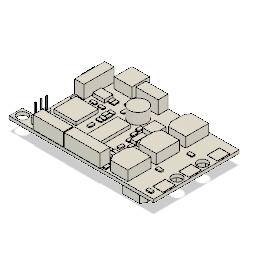
DIY_OneWheel_Frame (Autodesk Fusion 360 archive; units mm, degrees)
design "VESC-Fusion360"
Autodesk Fusion 360 part; units mm, degrees
sketch "Skizze1" plane through (0, 0, 0) normal (0, 1, 0) x (1, 0, 0)
  line L0 (65, 0) -> (65, -38.5) construction
  line L1 (65, -38.5) -> (0, -38.5) construction
  line L2 (6.3179, -1.8001) -> (10.6239, -1.8001)
  line L3 (10.6239, -1.8001) -> (10.6239, -15.3888)
  line L4 (10.6239, -15.3888) -> (6.3179, -15.3888)
  line L5 (6.3179, -15.3888) -> (6.3179, -1.8001)
  line L6 (16.7653, -8.6827) -> (18.1771, -8.6827)
  line L7 (18.1771, -8.6827) -> (18.1771, -11.0828)
  line L8 (18.1771, -11.0828) -> (16.7653, -11.0828)
  line L9 (16.7653, -11.0828) -> (16.7653, -8.6827)
  line L10 (18.3183, -8.6827) -> (19.7301, -8.6827)
  line L11 (19.7301, -8.6827) -> (19.7301, -11.0828)
  line L12 (19.7301, -11.0828) -> (18.3183, -11.0828)
  line L13 (18.3183, -11.0828) -> (18.3183, -8.6827)
  line L14 (21.8126, -6.2826) -> (23.2244, -6.2826)
  line L15 (23.2244, -6.2826) -> (23.2244, -8.6827)
  line L16 (23.2244, -8.6827) -> (21.8126, -8.6827)
  line L17 (21.8126, -8.6827) -> (21.8126, -6.2826)
  line L18 (23.9303, -7.412) -> (25.3421, -7.412)
  line L19 (25.3421, -7.412) -> (25.3421, -9.8121)
  line L20 (25.3421, -9.8121) -> (23.9303, -9.8121)
  line L21 (23.9303, -9.8121) -> (23.9303, -7.412)
  line L22 (23.9303, -9.9533) -> (25.3421, -9.9533)
  line L23 (25.3421, -9.9533) -> (25.3421, -12.3534)
  line L24 (25.3421, -12.3534) -> (23.9303, -12.3534)
  line L25 (23.9303, -12.3534) -> (23.9303, -9.9533)
  line L26 (12.8475, -13.8711) -> (15.2476, -13.8711)
  line L27 (15.2476, -13.8711) -> (15.2476, -15.177)
  line L28 (15.2476, -15.177) -> (12.8475, -15.177)
  line L29 (12.8475, -15.177) -> (12.8475, -13.8711)
  line L30 (16.5536, -13.9417) -> (18.9536, -13.9417)
  line L31 (18.9536, -13.9417) -> (18.9536, -15.2476)
  line L32 (18.9536, -15.2476) -> (16.5536, -15.2476)
  line L33 (16.5536, -15.2476) -> (16.5536, -13.9417)
  line L34 (20.8596, -13.8358) -> (23.2597, -13.8358)
  line L35 (23.2597, -13.8358) -> (23.2597, -15.1417)
  line L36 (23.2597, -15.1417) -> (20.8596, -15.1417)
  line L37 (20.8596, -15.1417) -> (20.8596, -13.8358)
  line L38 (20.6125, -15.2829) -> (22.0243, -15.2829)
  line L39 (22.0243, -15.2829) -> (22.0243, -17.683)
  line L40 (22.0243, -17.683) -> (20.6125, -17.683)
  line L41 (20.6125, -17.683) -> (20.6125, -15.2829)
  line L42 (22.2008, -15.2829) -> (23.5067, -15.2829)
  line L43 (23.5067, -15.2829) -> (23.5067, -17.683)
  line L44 (23.5067, -17.683) -> (22.2008, -17.683)
  line L45 (22.2008, -17.683) -> (22.2008, -15.2829)
  line L46 (21.1067, -17.8242) -> (23.5067, -17.8242)
  line L47 (23.5067, -17.8242) -> (23.5067, -19.236)
  line L48 (23.5067, -19.236) -> (21.1067, -19.236)
  line L49 (21.1067, -19.236) -> (21.1067, -17.8242)
  line L50 (21.142, -19.4125) -> (23.542, -19.4125)
  line L51 (23.542, -19.4125) -> (23.542, -20.7184)
  line L52 (23.542, -20.7184) -> (21.142, -20.7184)
  line L53 (21.142, -20.7184) -> (21.142, -19.4125)
  line L54 (21.6714, -22.8008) -> (22.9773, -22.8008)
  line L55 (22.9773, -22.8008) -> (22.9773, -25.2009)
  line L56 (22.9773, -25.2009) -> (21.6714, -25.2009)
  line L57 (21.6714, -25.2009) -> (21.6714, -22.8008)
  line L58 (7.2003, -15.6712) -> (8.5062, -15.6712)
  line L59 (8.5062, -15.6712) -> (8.5062, -18.0713)
  line L60 (8.5062, -18.0713) -> (7.2003, -18.0713)
  line L61 (7.2003, -18.0713) -> (7.2003, -15.6712)
  line L62 (17.683, -29.1893) -> (20.0831, -29.1893)
  line L63 (20.0831, -29.1893) -> (20.0831, -30.4952)
  line L64 (20.0831, -30.4952) -> (17.683, -30.4952)
  line L65 (17.683, -30.4952) -> (17.683, -29.1893)
  line L66 (22.4479, -29.9305) -> (23.7538, -29.9305)
  line L67 (23.7538, -29.9305) -> (23.7538, -32.3306)
  line L68 (23.7538, -32.3306) -> (22.4479, -32.3306)
  line L69 (22.4479, -32.3306) -> (22.4479, -29.9305)
  line L70 (14.7535, -32.5777) -> (17.1536, -32.5777)
  line L71 (17.1536, -32.5777) -> (17.1536, -33.9895)
  line L72 (17.1536, -33.9895) -> (14.7535, -33.9895)
  line L73 (14.7535, -33.9895) -> (14.7535, -32.5777)
  line L74 (17.33, -32.613) -> (19.7301, -32.613)
  line L75 (19.7301, -32.613) -> (19.7301, -33.9189)
  line L76 (19.7301, -33.9189) -> (17.33, -33.9189)
  line L77 (17.33, -33.9189) -> (17.33, -32.613)
  line L78 (26.7892, -31.3776) -> (31.8718, -31.3776)
  line L79 (31.8718, -31.3776) -> (31.8718, -33.6718)
  line L80 (31.8718, -33.6718) -> (26.7892, -33.6718)
  line L81 (26.7892, -33.6718) -> (26.7892, -31.3776)
  line L82 (35.6484, -28.5187) -> (36.9543, -28.5187)
  line L83 (36.9543, -28.5187) -> (36.9543, -30.9188)
  line L84 (36.9543, -30.9188) -> (35.6484, -30.9188)
  line L85 (35.6484, -30.9188) -> (35.6484, -28.5187)
  line L86 (35.6484, -31.307) -> (36.9543, -31.307)
  line L87 (36.9543, -31.307) -> (36.9543, -33.7071)
  line L88 (36.9543, -33.7071) -> (35.6484, -33.7071)
  line L89 (35.6484, -33.7071) -> (35.6484, -31.307)
  line L90 (37.1308, -28.1304) -> (39.5309, -28.1304)
  line L91 (39.5309, -28.1304) -> (39.5309, -29.5423)
  line L92 (39.5309, -29.5423) -> (37.1308, -29.5423)
  line L93 (37.1308, -29.5423) -> (37.1308, -28.1304)
  line L94 (37.1308, -29.6482) -> (39.5309, -29.6482)
  line L95 (39.5309, -29.6482) -> (39.5309, -31.06)
  line L96 (39.5309, -31.06) -> (37.1308, -31.06)
  line L97 (37.1308, -31.06) -> (37.1308, -29.6482)
  line L98 (37.1308, -31.1659) -> (39.5309, -31.1659)
  line L99 (39.5309, -31.1659) -> (39.5309, -32.5777)
  line L100 (39.5309, -32.5777) -> (37.1308, -32.5777)
  line L101 (37.1308, -32.5777) -> (37.1308, -31.1659)
  line L102 (37.1308, -32.7189) -> (39.5662, -32.7189)
  line L103 (39.5662, -32.7189) -> (39.5662, -34.1307)
  line L104 (39.5662, -34.1307) -> (37.1308, -34.1307)
  line L105 (37.1308, -34.1307) -> (37.1308, -32.7189)
  line L106 (41.4368, -35.366) -> (42.8486, -35.366)
  line L107 (42.8486, -35.366) -> (42.8486, -37.7661)
  line L108 (42.8486, -37.7661) -> (41.4368, -37.7661)
  line L109 (41.4368, -37.7661) -> (41.4368, -35.366)
  line L110 (36.8131, -24.4244) -> (38.1191, -24.4244)
  line L111 (38.1191, -24.4244) -> (38.1191, -26.8245)
  line L112 (38.1191, -26.8245) -> (36.8131, -26.8245)
  line L113 (36.8131, -26.8245) -> (36.8131, -24.4244)
  line L114 (38.9661, -22.0243) -> (40.2721, -22.0243)
  line L115 (40.2721, -22.0243) -> (40.2721, -24.4244)
  line L116 (40.2721, -24.4244) -> (38.9661, -24.4244)
  line L117 (38.9661, -24.4244) -> (38.9661, -22.0243)
  line L118 (36.1778, -19.7654) -> (37.4837, -19.7654)
  line L119 (37.4837, -19.7654) -> (37.4837, -22.1655)
  line L120 (37.4837, -22.1655) -> (36.1778, -22.1655)
  line L121 (36.1778, -22.1655) -> (36.1778, -19.7654)
  line L122 (34.9072, -16.6947) -> (36.2131, -16.6947)
  line L123 (36.2131, -16.6947) -> (36.2131, -19.0948)
  line L124 (36.2131, -19.0948) -> (34.9072, -19.0948)
  line L125 (34.9072, -19.0948) -> (34.9072, -16.6947)
  line L126 (34.0954, -13.377) -> (35.5072, -13.377)
  line L127 (35.5072, -13.377) -> (35.5072, -15.7771)
  line L128 (35.5072, -15.7771) -> (34.0954, -15.7771)
  line L129 (34.0954, -15.7771) -> (34.0954, -13.377)
  line L130 (37.8367, -16.5183) -> (40.1309, -16.5183)
  line L131 (40.1309, -16.5183) -> (40.1309, -21.6008)
  line L132 (40.1309, -21.6008) -> (37.8367, -21.6008)
  line L133 (37.8367, -21.6008) -> (37.8367, -16.5183)
  line L134 (40.378, -16.5183) -> (42.6722, -16.5183)
  line L135 (42.6722, -16.5183) -> (42.6722, -21.6008)
  line L136 (42.6722, -21.6008) -> (40.378, -21.6008)
  line L137 (40.378, -21.6008) -> (40.378, -16.5183)
  line L138 (55.0609, -12.2475) -> (57.4609, -12.2475)
  line L139 (57.4609, -12.2475) -> (57.4609, -13.6593)
  line L140 (57.4609, -13.6593) -> (55.0609, -13.6593)
  line L141 (55.0609, -13.6593) -> (55.0609, -12.2475)
  line L142 (53.8961, -25.2009) -> (56.2962, -25.2009)
  line L143 (56.2962, -25.2009) -> (56.2962, -26.6127)
  line L144 (56.2962, -26.6127) -> (53.8961, -26.6127)
  line L145 (53.8961, -26.6127) -> (53.8961, -25.2009)
  line L146 (60.0022, -35.6131) -> (62.4023, -35.6131)
  line L147 (62.4023, -35.6131) -> (62.4023, -37.0249)
  line L148 (62.4023, -37.0249) -> (60.0022, -37.0249)
  line L149 (60.0022, -37.0249) -> (60.0022, -35.6131)
  line L150 (11.3987, -31.323) -> (13.0958, -33.0201)
  line L151 (13.0958, -33.0201) -> (12.1724, -33.9435)
  line L152 (12.1724, -33.9435) -> (10.4753, -32.2464)
  line L153 (10.4753, -32.2464) -> (11.3987, -31.323)
  circle A0 centre (3.0001, -3.0001) radius 2.2942
  circle A1 centre (3.0001, -35.5072) radius 2.2942
  circle A2 centre (62.0493, -25.0245) radius 2.2942
  circle A3 centre (62.0493, -13.5181) radius 2.2942
  line L154 (59.9316, -16.483) -> (64.52, -16.483)
  line L155 (64.52, -16.483) -> (64.52, -22.0949)
  line L156 (64.52, -22.0949) -> (59.9316, -22.0949)
  line L157 (59.9316, -22.0949) -> (59.9316, -16.483)
  line L158 (59.9316, -3.7766) -> (64.52, -3.7766)
  line L159 (64.52, -3.7766) -> (64.52, -9.3886)
  line L160 (64.52, -9.3886) -> (59.9316, -9.3886)
  line L161 (59.9316, -9.3886) -> (59.9316, -3.7766)
  line L162 (59.9316, -28.201) -> (64.52, -28.201)
  line L163 (64.52, -28.201) -> (64.52, -33.813)
  line L164 (64.52, -33.813) -> (59.9316, -33.813)
  line L165 (59.9316, -33.813) -> (59.9316, -28.201)
  line L166 (26.1892, -15.9535) -> (32.1894, -15.9535)
  line L167 (32.1894, -15.9535) -> (32.1894, -30.9541)
  line L168 (32.1894, -30.9541) -> (26.1892, -30.9541)
  line L169 (26.1892, -30.9541) -> (26.1892, -15.9535)
  line L170 (10.9416, -34.3071) -> (24.5303, -34.3071)
  line L171 (24.5303, -34.3071) -> (24.5303, -38.6132)
  line L172 (24.5303, -38.6132) -> (10.9416, -38.6132)
  line L173 (10.9416, -38.6132) -> (10.9416, -34.3071)
  line L174 (8.9297, -17.33) -> (18.9536, -17.33)
  line L175 (18.9536, -17.33) -> (18.9536, -27.3539)
  line L176 (18.9536, -27.3539) -> (8.9297, -27.3539)
  line L177 (8.9297, -27.3539) -> (8.9297, -17.33)
  line L178 (11.2945, -8.4003) -> (16.6241, -8.4003)
  line L179 (16.6241, -8.4003) -> (16.6241, -12.2122)
  line L180 (16.6241, -12.2122) -> (11.2945, -12.2122)
  line L181 (11.2945, -12.2122) -> (11.2945, -8.4003)
  circle A4 centre (29.9658, -10.4121) radius 3.9884
  line L182 (36.5661, -9.5298) -> (41.6486, -9.5298)
  line L183 (41.6486, -9.5298) -> (41.6486, -15.1064)
  line L184 (41.6486, -15.1064) -> (36.5661, -15.1064)
  line L185 (36.5661, -15.1064) -> (36.5661, -9.5298)
  line L186 (13.1652, 3.5648) -> (21.1773, 3.5648)
  line L187 (21.1773, 3.5648) -> (21.1773, 0)
  line L188 (21.1773, 0) -> (13.1652, 0)
  line L189 (13.1652, 0) -> (13.1652, 3.5648)
  line L190 (9.1415, -34.0248) -> (8.0827, -34.0248)
  line L191 (8.0827, -34.0248) -> (7.3414, -34.8013)
  line L192 (7.3414, -34.8013) -> (7.3414, -35.8601)
  line L193 (7.3414, -35.8601) -> (8.0827, -36.6013)
  line L194 (8.0827, -36.6013) -> (9.1415, -36.6013)
  line L195 (9.1415, -36.6013) -> (9.8827, -35.8601)
  line L196 (9.8827, -35.8601) -> (9.8827, -34.8013)
  line L197 (9.8827, -34.8013) -> (9.1415, -34.0248)
  line L198 (9.1415, -31.4835) -> (8.0827, -31.4835)
  line L199 (8.0827, -31.4835) -> (7.3414, -32.2247)
  line L200 (7.3414, -32.2247) -> (7.3414, -33.2836)
  line L201 (7.3414, -33.2836) -> (8.0827, -34.0601)
  line L202 (8.0827, -34.0601) -> (9.1415, -34.0601)
  line L203 (9.1415, -34.0601) -> (9.8827, -33.2836)
  line L204 (9.8827, -33.2836) -> (9.8827, -32.2247)
  line L205 (9.8827, -32.2247) -> (9.1415, -31.4835)
  line L206 (9.1415, -28.9422) -> (8.0827, -28.9422)
  line L207 (8.0827, -28.9422) -> (7.3414, -29.6834)
  line L208 (7.3414, -29.6834) -> (7.3414, -30.7423)
  line L209 (7.3414, -30.7423) -> (8.0827, -31.4835)
  line L210 (8.0827, -31.4835) -> (9.1415, -31.4835)
  line L211 (9.1415, -31.4835) -> (9.8827, -30.7423)
  line L212 (9.8827, -30.7423) -> (9.8827, -29.6834)
  line L213 (9.8827, -29.6834) -> (9.1415, -28.9422)
  line L214 (8.365, -29.9658) -> (8.8591, -29.9658)
  line L215 (8.8591, -29.9658) -> (8.8591, -30.4599)
  line L216 (8.8591, -30.4599) -> (8.365, -30.4599)
  line L217 (8.365, -30.4599) -> (8.365, -29.9658)
  line L218 (8.365, -32.5071) -> (8.8591, -32.5071)
  line L219 (8.8591, -32.5071) -> (8.8591, -33.0012)
  line L220 (8.8591, -33.0012) -> (8.365, -33.0012)
  line L221 (8.365, -33.0012) -> (8.365, -32.5071)
  line L222 (8.365, -35.0483) -> (8.8591, -35.0483)
  line L223 (8.8591, -35.0483) -> (8.8591, -35.5425)
  line L224 (8.8591, -35.5425) -> (8.365, -35.5425)
  line L225 (8.365, -35.5425) -> (8.365, -35.0483)
  line L226 (0, 0) -> (0, -6.0002)
  line L227 (0, -6.0002) -> (6.0002, -6.0002)
  line L228 (6.0002, -6.0002) -> (6.0002, -32.5071)
  line L229 (6.0002, -32.5071) -> (0, -32.5071)
  line L230 (0, -32.5071) -> (0, -38.5073)
  line L231 (0, -38.5073) -> (65.0495, -38.5073)
  line L232 (65.0495, -38.5073) -> (65.0495, 0)
  line L233 (65.0495, 0) -> (0, 0)
  line L234 (43.2722, -3.4237) -> (43.2722, -9.0003)
  line L235 (43.2722, -9.0003) -> (44.5781, -11.4004)
  line L236 (44.5781, -11.4004) -> (52.3784, -11.4004)
  line L237 (52.3784, -11.4004) -> (52.3784, -1.0236)
  line L238 (52.3784, -1.0236) -> (44.5781, -1.0236)
  line L239 (44.5781, -1.0236) -> (43.2722, -3.4237)
  line L240 (43.2722, -16.6241) -> (43.2722, -22.2361)
  line L241 (43.2722, -22.2361) -> (44.5781, -24.6362)
  line L242 (44.5781, -24.6362) -> (52.3784, -24.6362)
  line L243 (52.3784, -24.6362) -> (52.3784, -14.2241)
  line L244 (52.3784, -14.2241) -> (44.5781, -14.2241)
  line L245 (44.5781, -14.2241) -> (43.2722, -16.6241)
  line L246 (43.2722, -29.4717) -> (43.2722, -35.0483)
  line L247 (43.2722, -35.0483) -> (44.5781, -37.4484)
  line L248 (44.5781, -37.4484) -> (52.3784, -37.4484)
  line L249 (52.3784, -37.4484) -> (52.3784, -27.0716)
  line L250 (52.3784, -27.0716) -> (44.5781, -27.0716)
  line L251 (44.5781, -27.0716) -> (43.2722, -29.4717)
  line L252 (24.9892, -34.1307) -> (41.0133, -34.1307)
  line L253 (41.0133, -34.1307) -> (41.0133, -38.6485)
  line L254 (41.0133, -38.6485) -> (24.9892, -38.6485)
  line L255 (24.9892, -38.6485) -> (24.9892, -34.1307)
  line L256 (23.295, -0.2471) -> (33.3189, -0.2471)
  line L257 (33.3189, -0.2471) -> (33.3189, -4.7649)
  line L258 (33.3189, -4.7649) -> (23.295, -4.7649)
  line L259 (23.295, -4.7649) -> (23.295, -0.2471)
  point P0 (-16.4157, 9.8589)
  point P1 (-16.4157, -22.6482)
  point P2 (35.1631, 11.9797)
  point P3 (-5.3762, 16.1231)
  point P4 (5.2943, -3.0001)
  point P5 (5.2943, -35.5072)
  point P6 (64.3435, -25.0245)
  point P7 (64.3435, -13.5181)
  point P8 (33.9542, -10.4121)
extrude "Extrusion1" add sketch "Skizze1" against normal blind 1.5 contours L2 L3 L4 L5 | L6 L7 L8 L9 | L10 L11 L12 L13 | L14 L15 L16 L17 | L18 L19 L20 L21 | L22 L23 L24 L25 | L26 L27 L28 L29 | L30 L31 L32 L33 | L34 L35 L36 L37 | L38 L39 L40 L41 | L42 L43 L44 L45 | L46 L47 L48 L49 | L50 L51 L52 L53 | L54 L55 L56 L57 | L58 L59 L60 L61 | L62 L63 L64 L65 | L66 L67 L68 L69 | L70 L71 L72 L73 | L74 L75 L76 L77 | L78 L79 L80 L81 | L82 L83 L84 L85 | L86 L87 L88 L89 | L90 L91 L92 L93 | L94 L95 L96 L97 | L98 L99 L100 L101 | L102 L103 L105 L170 L171 L173 L188 L226 L227 L228 L229 L230 L231 L232 L233 L252 L253 L255 | L102 L103 L104 L105 L252 | L104 L231 L252 L253 L255 | L170 L171 L173 L231 | L106 L107 L108 L109 | L110 L111 L112 L113 | L114 L115 L116 L117 | L118 L119 L120 L121 | L122 L123 L124 L125 | L126 L127 L128 L129 | L130 L131 L132 L133 | L134 L135 L136 L137 | L138 L139 L140 L141 | L142 L143 L144 L145 | L146 L147 L148 L149 | L150 L151 L152 L153 | L154 L155 L156 L157 | L158 L159 L160 L161 | L162 L163 L164 L165 | L166 L167 L168 L169 | L174 L175 L176 L177 | L178 L179 L180 L181 | A4 | L182 L183 L184 L185 | L190 L191 L197 L201 L202 L203 | L190 L191 L197 L198 L199 L200 L201 L203 L204 L205 L210 | L191 L192 L193 L194 L195 L196 L197 L201 L202 L203 | L198 L206 L207 L208 L209 L210 L211 L212 L213 | L214 L215 L216 L217 | L218 L219 L220 L221 | L222 L223 L224 L225 | L234 L235 L236 L237 L238 L239 | L240 L241 L242 L243 L244 L245 | L246 L247 L248 L249 L250 L251 | L256 L257 L258 L259
extrude "Extrusion2" add sketch "Skizze1" along normal blind 6 contours L2 L3 L4 L5 | L104 L231 L252 L253 L255 | L231 L253 L254 L255 | L170 L171 L173 L231 | L171 L172 L173 L231 | L256 L257 L258 L259
extrude "Extrusion3" add sketch "Skizze1" along normal blind 4.5 contours L234 L235 L236 L237 L238 L239 | L240 L241 L242 L243 L244 L245 | L246 L247 L248 L249 L250 L251
extrude "Extrusion4" add sketch "Skizze1" along normal blind 5 contours A4
extrude "Extrusion5" add sketch "Skizze1" along normal blind 1.5 contours L178 L179 L180 L181
extrude "Extrusion6" add sketch "Skizze1" along normal blind 1.5 contours L166 L167 L168 L169 | L174 L175 L176 L177
extrude "Extrusion7" add sketch "Skizze1" along normal blind 2 contours L182 L183 L184 L185
extrude "Extrusion8" add sketch "Skizze1" along normal blind 1.5 contours L78 L79 L80 L81 | L130 L131 L132 L133 | L134 L135 L136 L137
extrude "Extrusion9" add sketch "Skizze1" along normal blind 0.5 contours L6 L7 L8 L9 | L10 L11 L12 L13 | L14 L15 L16 L17 | L18 L19 L20 L21 | L22 L23 L24 L25 | L26 L27 L28 L29 | L30 L31 L32 L33 | L34 L35 L36 L37 | L38 L39 L40 L41 | L42 L43 L44 L45 | L46 L47 L48 L49 | L50 L51 L52 L53 | L54 L55 L56 L57 | L58 L59 L60 L61 | L62 L63 L64 L65 | L66 L67 L68 L69 | L70 L71 L72 L73 | L74 L75 L76 L77 | L82 L83 L84 L85 | L86 L87 L88 L89 | L90 L91 L92 L93 | L94 L95 L96 L97 | L98 L99 L100 L101 | L102 L103 L104 L105 L252 | L106 L107 L108 L109 | L110 L111 L112 L113 | L114 L115 L116 L117 | L118 L119 L120 L121 | L122 L123 L124 L125 | L126 L127 L128 L129 | L138 L139 L140 L141 | L142 L143 L144 L145 | L146 L147 L148 L149 | L150 L151 L152 L153
extrude "Extrusion11" add sketch "Skizze1" along normal blind 2.5 contours L190 L191 L197 L201 L202 L203 | L190 L191 L197 L198 L199 L200 L201 L203 L204 L205 L210 | L191 L192 L193 L194 L195 L196 L197 L201 L202 L203 | L198 L206 L207 L208 L209 L210 L211 L212 L213
extrude "Extrusion21" add 3 faces at (8.5297, 0, 30.2952) (8.5297, 0, 32.8365) (8.6944, 0, 35.3778) along direction (0, 1, 0) blind 8
sketch "Skizze5" plane through (0, 0, 0) normal (0, 1, 0) x (1, 0, 0)
  line L0 (13.1652, 3.5648) -> (21.1773, 3.5648)
  line L1 (21.1773, 3.5648) -> (21.1773, -4.4352)
  line L2 (21.1773, -4.4352) -> (13.1652, -4.4352)
  line L3 (13.1652, -4.4352) -> (13.1652, 3.5648)
  point P0 (13.1652, 3.5648)
  point P1 (21.1773, 3.5648)
  dimension "d61" = 8
  constraint horizontal L0
  constraint vertical L1
  constraint horizontal L2
  constraint vertical L3
  constraint coincident P0 L0.start
  constraint coincident P1 L0.end
  measures "d61" distance of P0 L2.end
extrude "Extrusion12" add sketch "Skizze5" along normal blind 4.75
sketch "Skizze4" plane through (0, 0, 0) normal (0, 1, 0) x (1, 0, 0)
  line L0 (10.518, -29.6834) -> (13.3064, -29.6834)
  line L1 (13.3064, -29.6834) -> (13.3064, -34.0954)
  line L2 (13.3064, -34.0954) -> (10.518, -34.0954)
  line L3 (10.518, -34.0954) -> (10.518, -29.6834)
  line L4 (11.471, -27.2481) -> (13.8711, -27.2481)
  line L5 (13.8711, -27.2481) -> (13.8711, -28.6599)
  line L6 (13.8711, -28.6599) -> (11.471, -28.6599)
  line L7 (11.471, -28.6599) -> (11.471, -27.2481)
  line L8 (10.4827, -24.3185) -> (11.7887, -24.3185)
  line L9 (11.7887, -24.3185) -> (11.7887, -26.7186)
  line L10 (11.7887, -26.7186) -> (10.4827, -26.7186)
  line L11 (10.4827, -26.7186) -> (10.4827, -24.3185)
  line L12 (13.5534, -20.6478) -> (14.8594, -20.6478)
  line L13 (14.8594, -20.6478) -> (14.8594, -23.0479)
  line L14 (14.8594, -23.0479) -> (13.5534, -23.0479)
  line L15 (13.5534, -23.0479) -> (13.5534, -20.6478)
  line L16 (13.5534, -17.8595) -> (14.8594, -17.8595)
  line L17 (14.8594, -17.8595) -> (14.8594, -20.2596)
  line L18 (14.8594, -20.2596) -> (13.5534, -20.2596)
  line L19 (13.5534, -20.2596) -> (13.5534, -17.8595)
  line L20 (9.8121, -17.9301) -> (13.024, -17.9301)
  line L21 (13.024, -17.9301) -> (13.024, -22.942)
  line L22 (13.024, -22.942) -> (9.8121, -22.942)
  line L23 (9.8121, -22.942) -> (9.8121, -17.9301)
  line L24 (8.5768, -14.7888) -> (9.8827, -14.7888)
  line L25 (9.8827, -14.7888) -> (9.8827, -17.1889)
  line L26 (9.8827, -17.1889) -> (8.5768, -17.1889)
  line L27 (8.5768, -17.1889) -> (8.5768, -14.7888)
  line L28 (9.4239, -13.2711) -> (11.824, -13.2711)
  line L29 (11.824, -13.2711) -> (11.824, -14.6829)
  line L30 (11.824, -14.6829) -> (9.4239, -14.6829)
  line L31 (9.4239, -14.6829) -> (9.4239, -13.2711)
  line L32 (9.4239, -11.7534) -> (11.824, -11.7534)
  line L33 (11.824, -11.7534) -> (11.824, -13.1652)
  line L34 (11.824, -13.1652) -> (9.4239, -13.1652)
  line L35 (9.4239, -13.1652) -> (9.4239, -11.7534)
  line L36 (9.4239, -10.2004) -> (11.824, -10.2004)
  line L37 (11.824, -10.2004) -> (11.824, -11.6122)
  line L38 (11.824, -11.6122) -> (9.4239, -11.6122)
  line L39 (9.4239, -11.6122) -> (9.4239, -10.2004)
  line L40 (9.4239, -8.6827) -> (11.824, -8.6827)
  line L41 (11.824, -8.6827) -> (11.824, -10.0945)
  line L42 (11.824, -10.0945) -> (9.4239, -10.0945)
  line L43 (9.4239, -10.0945) -> (9.4239, -8.6827)
  line L44 (9.4239, -7.165) -> (11.824, -7.165)
  line L45 (11.824, -7.165) -> (11.824, -8.5768)
  line L46 (11.824, -8.5768) -> (9.4239, -8.5768)
  line L47 (9.4239, -8.5768) -> (9.4239, -7.165)
  line L48 (12.0004, -7.2003) -> (14.4005, -7.2003)
  line L49 (14.4005, -7.2003) -> (14.4005, -8.5062)
  line L50 (14.4005, -8.5062) -> (12.0004, -8.5062)
  line L51 (12.0004, -8.5062) -> (12.0004, -7.2003)
  line L52 (12.0004, -11.7534) -> (14.4005, -11.7534)
  line L53 (14.4005, -11.7534) -> (14.4005, -13.0593)
  line L54 (14.4005, -13.0593) -> (12.0004, -13.0593)
  line L55 (12.0004, -13.0593) -> (12.0004, -11.7534)
  line L56 (11.9651, -13.3064) -> (14.3652, -13.3064)
  line L57 (14.3652, -13.3064) -> (14.3652, -14.6123)
  line L58 (14.3652, -14.6123) -> (11.9651, -14.6123)
  line L59 (11.9651, -14.6123) -> (11.9651, -13.3064)
  line L60 (9.4239, -5.6473) -> (11.824, -5.6473)
  line L61 (11.824, -5.6473) -> (11.824, -7.0591)
  line L62 (11.824, -7.0591) -> (9.4239, -7.0591)
  line L63 (9.4239, -7.0591) -> (9.4239, -5.6473)
  line L64 (9.4239, -4.1296) -> (11.824, -4.1296)
  line L65 (11.824, -4.1296) -> (11.824, -5.5414)
  line L66 (11.824, -5.5414) -> (9.4239, -5.5414)
  line L67 (9.4239, -5.5414) -> (9.4239, -4.1296)
  line L68 (11.471, -3.3531) -> (13.8711, -3.3531) construction
  line L69 (13.8711, -3.3531) -> (13.8711, -4.7649) construction
  line L70 (13.8711, -4.7649) -> (11.471, -4.7649) construction
  line L71 (11.471, -4.7649) -> (11.471, -3.3531) construction
  line L72 (15.2829, -9.0709) -> (17.683, -9.0709) construction
  line L73 (17.683, -9.0709) -> (17.683, -10.4827) construction
  line L74 (17.683, -10.4827) -> (15.2829, -10.4827) construction
  line L75 (15.2829, -10.4827) -> (15.2829, -9.0709) construction
  line L76 (16.8006, -9.0709) -> (19.2007, -9.0709) construction
  line L77 (19.2007, -9.0709) -> (19.2007, -10.4827) construction
  line L78 (19.2007, -10.4827) -> (16.8006, -10.4827) construction
  line L79 (16.8006, -10.4827) -> (16.8006, -9.0709) construction
  line L80 (18.3536, -9.0709) -> (20.7537, -9.0709) construction
  line L81 (20.7537, -9.0709) -> (20.7537, -10.4827) construction
  line L82 (20.7537, -10.4827) -> (18.3536, -10.4827) construction
  line L83 (18.3536, -10.4827) -> (18.3536, -9.0709) construction
  line L84 (18.7419, -13.5181) -> (21.142, -13.5181) construction
  line L85 (21.142, -13.5181) -> (21.142, -14.93) construction
  line L86 (21.142, -14.93) -> (18.7419, -14.93) construction
  line L87 (18.7419, -14.93) -> (18.7419, -13.5181) construction
  line L88 (17.2595, -13.5181) -> (19.6595, -13.5181) construction
  line L89 (19.6595, -13.5181) -> (19.6595, -14.93)
  line L90 (19.6595, -14.93) -> (17.2595, -14.93) construction
  line L91 (17.2595, -14.93) -> (17.2595, -13.5181) construction
  line L92 (15.7418, -13.5181) -> (18.1418, -13.5181) construction
  line L93 (18.1418, -13.5181) -> (18.1418, -14.93) construction
  line L94 (18.1418, -14.93) -> (15.7418, -14.93) construction
  line L95 (15.7418, -14.93) -> (15.7418, -13.5181) construction
  line L96 (14.5064, -1.0589) -> (16.9065, -1.0589)
  line L97 (16.9065, -1.0589) -> (16.9065, -2.4707)
  line L98 (16.9065, -2.4707) -> (14.5064, -2.4707)
  line L99 (14.5064, -2.4707) -> (14.5064, -1.0589)
  line L100 (9.4239, -2.6472) -> (11.824, -2.6472)
  line L101 (11.824, -2.6472) -> (11.824, -3.9531)
  line L102 (11.824, -3.9531) -> (9.4239, -3.9531)
  line L103 (9.4239, -3.9531) -> (9.4239, -2.6472)
  line L104 (18.9536, -18.5301) -> (21.3537, -18.5301)
  line L105 (21.3537, -18.5301) -> (21.3537, -19.836)
  line L106 (21.3537, -19.836) -> (18.9536, -19.836)
  line L107 (18.9536, -19.836) -> (18.9536, -18.5301)
  line L108 (18.9536, -16.8712) -> (21.3537, -16.8712)
  line L109 (21.3537, -16.8712) -> (21.3537, -18.1771)
  line L110 (21.3537, -18.1771) -> (18.9536, -18.1771)
  line L111 (18.9536, -18.1771) -> (18.9536, -16.8712)
  line L112 (22.6597, -14.5417) -> (24.0715, -14.5417)
  line L113 (24.0715, -14.5417) -> (24.0715, -16.9418)
  line L114 (24.0715, -16.9418) -> (22.6597, -16.9418)
  line L115 (22.6597, -16.9418) -> (22.6597, -14.5417)
  line L116 (25.2362, -15.1064) -> (27.5304, -15.1064)
  line L117 (27.5304, -15.1064) -> (27.5304, -20.189)
  line L118 (27.5304, -20.189) -> (25.2362, -20.189)
  line L119 (25.2362, -20.189) -> (25.2362, -15.1064)
  line L120 (27.6716, -15.1064) -> (29.9658, -15.1064)
  line L121 (29.9658, -15.1064) -> (29.9658, -20.189)
  line L122 (29.9658, -20.189) -> (27.6716, -20.189)
  line L123 (27.6716, -20.189) -> (27.6716, -15.1064)
  line L124 (24.2127, -21.2831) -> (25.5186, -21.2831)
  line L125 (25.5186, -21.2831) -> (25.5186, -23.6832)
  line L126 (25.5186, -23.6832) -> (24.2127, -23.6832)
  line L127 (24.2127, -23.6832) -> (24.2127, -21.2831)
  line L128 (17.7889, -32.9306) -> (20.189, -32.9306)
  line L129 (20.189, -32.9306) -> (20.189, -34.3424)
  line L130 (20.189, -34.3424) -> (17.7889, -34.3424)
  line L131 (17.7889, -34.3424) -> (17.7889, -32.9306)
  line L132 (15.3605, -32.2186) -> (17.0576, -33.9157)
  line L133 (17.0576, -33.9157) -> (16.1341, -34.8391)
  line L134 (16.1341, -34.8391) -> (14.437, -33.142)
  line L135 (14.437, -33.142) -> (15.3605, -32.2186)
  line L136 (17.7889, -31.4129) -> (20.189, -31.4129)
  line L137 (20.189, -31.4129) -> (20.189, -32.8247)
  line L138 (20.189, -32.8247) -> (17.7889, -32.8247)
  line L139 (17.7889, -32.8247) -> (17.7889, -31.4129)
  line L140 (17.7889, -29.9305) -> (20.189, -29.9305)
  line L141 (20.189, -29.9305) -> (20.189, -31.3423)
  line L142 (20.189, -31.3423) -> (17.7889, -31.3423)
  line L143 (17.7889, -31.3423) -> (17.7889, -29.9305)
  line L144 (17.8242, -28.4834) -> (20.2243, -28.4834)
  line L145 (20.2243, -28.4834) -> (20.2243, -29.754)
  line L146 (20.2243, -29.754) -> (17.8242, -29.754)
  line L147 (17.8242, -29.754) -> (17.8242, -28.4834)
  line L148 (21.0008, -28.3069) -> (23.4009, -28.3069)
  line L149 (23.4009, -28.3069) -> (23.4009, -29.5776)
  line L150 (23.4009, -29.5776) -> (21.0008, -29.5776)
  line L151 (21.0008, -29.5776) -> (21.0008, -28.3069)
  line L152 (21.0008, -26.7892) -> (23.4009, -26.7892)
  line L153 (23.4009, -26.7892) -> (23.4009, -28.0952)
  line L154 (23.4009, -28.0952) -> (21.0008, -28.0952)
  line L155 (21.0008, -28.0952) -> (21.0008, -26.7892)
  line L156 (20.9655, -32.9659) -> (22.6597, -32.9659)
  line L157 (22.6597, -32.9659) -> (22.6597, -33.8483)
  line L158 (22.6597, -33.8483) -> (20.9655, -33.8483)
  line L159 (20.9655, -33.8483) -> (20.9655, -32.9659)
  line L160 (20.9655, -31.5188) -> (22.6597, -31.5188)
  line L161 (22.6597, -31.5188) -> (22.6597, -32.4012)
  line L162 (22.6597, -32.4012) -> (20.9655, -32.4012)
  line L163 (20.9655, -32.4012) -> (20.9655, -31.5188)
  line L164 (20.9655, -30.107) -> (22.6597, -30.107)
  line L165 (22.6597, -30.107) -> (22.6597, -30.9894)
  line L166 (22.6597, -30.9894) -> (20.9655, -30.9894)
  line L167 (20.9655, -30.9894) -> (20.9655, -30.107)
  line L168 (24.3538, -29.4717) -> (29.9305, -29.4717)
  line L169 (29.9305, -29.4717) -> (29.9305, -34.5542)
  line L170 (29.9305, -34.5542) -> (24.3538, -34.5542)
  line L171 (24.3538, -34.5542) -> (24.3538, -29.4717)
  line L172 (27.5657, -23.1538) -> (29.8599, -23.1538)
  line L173 (29.8599, -23.1538) -> (29.8599, -28.2363)
  line L174 (29.8599, -28.2363) -> (27.5657, -28.2363)
  line L175 (27.5657, -28.2363) -> (27.5657, -23.1538)
  line L176 (32.1188, -26.1539) -> (34.413, -26.1539)
  line L177 (34.413, -26.1539) -> (34.413, -31.2364)
  line L178 (34.413, -31.2364) -> (32.1188, -31.2364)
  line L179 (32.1188, -31.2364) -> (32.1188, -26.1539)
  line L180 (34.9072, -22.9773) -> (41.5074, -22.9773)
  line L181 (41.5074, -22.9773) -> (41.5074, -29.8246)
  line L182 (41.5074, -29.8246) -> (34.9072, -29.8246)
  line L183 (34.9072, -29.8246) -> (34.9072, -22.9773)
  line L184 (31.5894, -12.9534) -> (33.8836, -12.9534)
  line L185 (33.8836, -12.9534) -> (33.8836, -18.036)
  line L186 (33.8836, -18.036) -> (31.5894, -18.036)
  line L187 (31.5894, -18.036) -> (31.5894, -12.9534)
  line L188 (36.5661, -16.73) -> (42.178, -16.73)
  line L189 (42.178, -16.73) -> (42.178, -21.3184)
  line L190 (42.178, -21.3184) -> (36.5661, -21.3184)
  line L191 (36.5661, -21.3184) -> (36.5661, -16.73)
  line L192 (35.1542, -8.2591) -> (41.7545, -8.2591)
  line L193 (41.7545, -8.2591) -> (41.7545, -15.1064)
  line L194 (41.7545, -15.1064) -> (35.1542, -15.1064)
  line L195 (35.1542, -15.1064) -> (35.1542, -8.2591)
  line L196 (34.1307, -0.8471) -> (39.7426, -0.8471)
  line L197 (39.7426, -0.8471) -> (39.7426, -5.4355)
  line L198 (39.7426, -5.4355) -> (34.1307, -5.4355)
  line L199 (34.1307, -5.4355) -> (34.1307, -0.8471)
  line L200 (42.9898, -12.0004) -> (45.3899, -12.0004)
  line L201 (45.3899, -12.0004) -> (45.3899, -13.4123)
  line L202 (45.3899, -13.4123) -> (42.9898, -13.4123)
  line L203 (42.9898, -13.4123) -> (42.9898, -12.0004)
  line L204 (45.7782, -12.0004) -> (48.1782, -12.0004)
  line L205 (48.1782, -12.0004) -> (48.1782, -13.4123)
  line L206 (48.1782, -13.4123) -> (45.7782, -13.4123)
  line L207 (45.7782, -13.4123) -> (45.7782, -12.0004)
  line L208 (14.7888, -6.0002) -> (17.1889, -6.0002)
  line L209 (17.1889, -6.0002) -> (17.1889, -7.412)
  line L210 (17.1889, -7.412) -> (14.7888, -7.412)
  line L211 (14.7888, -7.412) -> (14.7888, -6.0002)
  line L212 (16.0594, -4.5531) -> (18.4595, -4.5531)
  line L213 (18.4595, -4.5531) -> (18.4595, -5.859)
  line L214 (18.4595, -5.859) -> (16.0594, -5.859)
  line L215 (16.0594, -5.859) -> (16.0594, -4.5531)
  line L216 (17.7183, -6.0002) -> (20.1184, -6.0002)
  line L217 (20.1184, -6.0002) -> (20.1184, -7.412)
  line L218 (20.1184, -7.412) -> (17.7183, -7.412)
  line L219 (17.7183, -7.412) -> (17.7183, -6.0002)
  line L220 (20.8596, -5.9296) -> (23.2597, -5.9296)
  line L221 (23.2597, -5.9296) -> (23.2597, -7.2356)
  line L222 (23.2597, -7.2356) -> (20.8596, -7.2356)
  line L223 (20.8596, -7.2356) -> (20.8596, -5.9296)
  line L224 (19.5184, -0.4941) -> (23.0832, -0.4941)
  line L225 (23.0832, -0.4941) -> (23.0832, -3.2825)
  line L226 (23.0832, -3.2825) -> (19.5184, -3.2825)
  line L227 (19.5184, -3.2825) -> (19.5184, -0.4941)
  line L228 (24.9186, -3.106) -> (28.4834, -3.106)
  line L229 (28.4834, -3.106) -> (28.4834, -5.8943)
  line L230 (28.4834, -5.8943) -> (24.9186, -5.8943)
  line L231 (24.9186, -5.8943) -> (24.9186, -3.106)
  line L232 (42.4604, -25.2009) -> (44.8605, -25.2009)
  line L233 (44.8605, -25.2009) -> (44.8605, -26.6127)
  line L234 (44.8605, -26.6127) -> (42.4604, -26.6127)
  line L235 (42.4604, -26.6127) -> (42.4604, -25.2009)
  line L236 (45.0017, -25.2009) -> (47.4017, -25.2009)
  line L237 (47.4017, -25.2009) -> (47.4017, -26.6127)
  line L238 (47.4017, -26.6127) -> (45.0017, -26.6127)
  line L239 (45.0017, -26.6127) -> (45.0017, -25.2009)
  line L240 (47.6841, -25.2009) -> (50.0842, -25.2009)
  line L241 (50.0842, -25.2009) -> (50.0842, -26.6127)
  line L242 (50.0842, -26.6127) -> (47.6841, -26.6127)
  line L243 (47.6841, -26.6127) -> (47.6841, -25.2009)
  line L244 (41.1898, -34.3424) -> (42.6016, -34.3424)
  line L245 (42.6016, -34.3424) -> (42.6016, -36.7425)
  line L246 (42.6016, -36.7425) -> (41.1898, -36.7425)
  line L247 (41.1898, -36.7425) -> (41.1898, -34.3424)
  line L248 (49.8371, -11.5416) -> (57.6374, -11.5416)
  line L249 (57.6374, -11.5416) -> (58.9433, -9.1415)
  line L250 (58.9433, -9.1415) -> (58.9433, -3.5295)
  line L251 (58.9433, -3.5295) -> (57.6374, -1.1295)
  line L252 (57.6374, -1.1295) -> (49.8371, -1.1295)
  line L253 (49.8371, -1.1295) -> (49.8371, -11.5416)
  line L254 (49.8371, -14.2241) -> (57.6374, -14.2241)
  line L255 (57.6374, -14.2241) -> (58.9433, -16.6241)
  line L256 (58.9433, -16.6241) -> (58.9433, -22.2361)
  line L257 (58.9433, -22.2361) -> (57.6374, -24.6362)
  line L258 (57.6374, -24.6362) -> (49.8371, -24.6362)
  line L259 (49.8371, -24.6362) -> (49.8371, -14.2241)
  line L260 (49.8371, -37.4484) -> (57.6374, -37.4484)
  line L261 (57.6374, -37.4484) -> (58.9433, -35.0483)
  line L262 (58.9433, -35.0483) -> (58.9433, -29.4717)
  line L263 (58.9433, -29.4717) -> (57.6374, -27.0716)
  line L264 (57.6374, -27.0716) -> (49.8371, -27.0716)
  line L265 (49.8371, -27.0716) -> (49.8371, -37.4484)
  line L266 (0, -38.5073) -> (0, -32.5071)
  line L267 (0, -32.5071) -> (6.0002, -32.5071)
  line L268 (6.0002, -32.5071) -> (6.0002, -6.0002)
  line L269 (6.0002, -6.0002) -> (0, -6.0002)
  line L270 (0, -6.0002) -> (0, 0)
  line L271 (0, 0) -> (65.0495, 0)
  line L272 (65.0495, 0) -> (65.0495, -38.5073)
  line L273 (65.0495, -38.5073) -> (0, -38.5073)
  line L274 (23.3303, -6.1767) -> (29.9305, -6.1767)
  line L275 (29.9305, -6.1767) -> (29.9305, -13.024)
  line L276 (29.9305, -13.024) -> (23.3303, -13.024)
  line L277 (23.3303, -13.024) -> (23.3303, -6.1767)
  line L278 (12.6711, -4.7649) -> (12.6711, -3.3531) construction
  line L279 (13.8711, -4.059) -> (11.471, -4.059) construction
  line L280 (15.2829, -9.7768) -> (20.7537, -9.7768) construction
  line L281 (16.483, -10.4827) -> (16.483, -9.0709) construction
  line L282 (18.0007, -10.4827) -> (18.0007, -9.0709) construction
  line L283 (19.5537, -10.4827) -> (19.5537, -9.0709) construction
  line L284 (16.9418, -14.93) -> (16.9418, -13.5181) construction
  line L285 (18.4595, -14.93) -> (18.4595, -13.5181) construction
  line L286 (19.9419, -14.93) -> (19.9419, -13.5181) construction
  line L287 (21.142, -14.2241) -> (15.7418, -14.2241) construction
  line L288 (13.3711, -2.859) -> (11.9711, -2.859)
  line L289 (11.9711, -2.859) -> (11.9711, -5.259)
  line L290 (11.9711, -5.259) -> (13.3711, -5.259)
  line L291 (13.3711, -5.259) -> (13.3711, -2.859)
  line L292 (13.3711, -2.859) -> (11.9711, -5.259) construction
  line L293 (11.9711, -2.859) -> (13.3711, -5.259) construction
  line L294 (17.183, -8.5768) -> (15.783, -8.5768)
  line L295 (15.783, -8.5768) -> (15.783, -10.9768)
  line L296 (15.783, -10.9768) -> (17.183, -10.9768)
  line L297 (17.183, -10.9768) -> (17.183, -8.5768)
  line L298 (17.183, -8.5768) -> (15.783, -10.9768) construction
  line L299 (15.783, -8.5768) -> (17.183, -10.9768) construction
  line L300 (18.7007, -8.5768) -> (17.3007, -8.5768)
  line L301 (17.3007, -8.5768) -> (17.3007, -10.9768)
  line L302 (17.3007, -10.9768) -> (18.7007, -10.9768)
  line L303 (18.7007, -10.9768) -> (18.7007, -8.5768)
  line L304 (18.7007, -8.5768) -> (17.3007, -10.9768) construction
  line L305 (17.3007, -8.5768) -> (18.7007, -10.9768) construction
  line L306 (20.2537, -8.5768) -> (18.8537, -8.5768)
  line L307 (18.8537, -8.5768) -> (18.8537, -10.9768)
  line L308 (18.8537, -10.9768) -> (20.2537, -10.9768)
  line L309 (20.2537, -10.9768) -> (20.2537, -8.5768)
  line L310 (20.2537, -8.5768) -> (18.8537, -10.9768) construction
  line L311 (18.8537, -8.5768) -> (20.2537, -10.9768) construction
  line L312 (17.6418, -15.4241) -> (16.2418, -15.4241)
  line L313 (16.2418, -15.4241) -> (16.2418, -13.0241)
  line L314 (16.2418, -13.0241) -> (17.6418, -13.0241)
  line L315 (17.6418, -13.0241) -> (17.6418, -15.4241)
  line L316 (17.6418, -15.4241) -> (16.2418, -13.0241) construction
  line L317 (16.2418, -15.4241) -> (17.6418, -13.0241) construction
  line L318 (19.1595, -13.0241) -> (17.7595, -13.0241)
  line L319 (17.7595, -13.0241) -> (17.7595, -15.4241)
  line L320 (17.7595, -15.4241) -> (19.1595, -15.4241)
  line L321 (19.1595, -15.4241) -> (19.1595, -13.0241)
  line L322 (19.1595, -13.0241) -> (17.7595, -15.4241) construction
  line L323 (17.7595, -13.0241) -> (19.1595, -15.4241) construction
  line L324 (20.6419, -13.0241) -> (19.2419, -13.0241)
  line L325 (19.2419, -13.0241) -> (19.2419, -15.4241)
  line L326 (19.2419, -15.4241) -> (20.6419, -15.4241)
  line L327 (20.6419, -15.4241) -> (20.6419, -13.0241)
  line L328 (20.6419, -13.0241) -> (19.2419, -15.4241) construction
  line L329 (19.2419, -13.0241) -> (20.6419, -15.4241) construction
  point P0 (12.6711, -4.059)
  point P1 (16.483, -9.7768)
  point P2 (18.0007, -9.7768)
  point P3 (19.5537, -9.7768)
  point P4 (16.9418, -14.2241)
  point P5 (18.4595, -14.2241)
  point P6 (19.9419, -14.2241)
  dimension "d62" = 1.4
  dimension "d63" = 2.4
  dimension "d64" = 2.4
  dimension "d65" = 1.4
  dimension "d66" = 1.4
  dimension "d67" = 2.4
  dimension "d68" = 2.4
  dimension "d69" = 1.4
  dimension "d70" = 2.4
  dimension "d71" = 1.4
  dimension "d72" = 2.4
  dimension "d73" = 1.4
  dimension "d74" = 1.4
  dimension "d75" = 2.4
  constraint midpoint L70 L278.start
  constraint midpoint L68 L278.end
  constraint midpoint L69 L279.start
  constraint midpoint L71 L279.end
  constraint midpoint L75 L280.start
  constraint midpoint L81 L280.end
  constraint midpoint L74 L281.start
  constraint midpoint L72 L281.end
  constraint midpoint L78 L282.start
  constraint midpoint L76 L282.end
  constraint midpoint L82 L283.start
  constraint midpoint L80 L283.end
  constraint midpoint L94 L284.start
  constraint midpoint L92 L284.end
  constraint midpoint L90 L285.start
  constraint midpoint L88 L285.end
  constraint midpoint L86 L286.start
  constraint midpoint L84 L286.end
  constraint midpoint L85 L287.start
  constraint midpoint L95 L287.end
  constraint perpendicular L288 L289
  constraint parallel L288 L290
  constraint parallel L289 L291
  constraint horizontal L288
  constraint coincident L292 P0
  constraint coincident L293 P0
  constraint midpoint L278 P0
  constraint perpendicular L294 L295
  constraint parallel L294 L296
  constraint parallel L295 L297
  constraint horizontal L294
  constraint coincident L298 P1
  constraint coincident L299 P1
  constraint midpoint L281 P1
  constraint perpendicular L300 L301
  constraint parallel L300 L302
  constraint parallel L301 L303
  constraint horizontal L300
  constraint coincident L304 P2
  constraint coincident L305 P2
  constraint midpoint L282 P2
  constraint perpendicular L306 L307
  constraint parallel L306 L308
  constraint parallel L307 L309
  constraint horizontal L306
  constraint coincident L310 P3
  constraint coincident L311 P3
  constraint midpoint L283 P3
  constraint perpendicular L312 L313
  constraint parallel L312 L314
  constraint parallel L313 L315
  constraint horizontal L312
  constraint coincident L316 P4
  constraint coincident L317 P4
  constraint midpoint L284 P4
  constraint perpendicular L318 L319
  constraint parallel L318 L320
  constraint parallel L319 L321
  constraint horizontal L318
  constraint coincident L322 P5
  constraint coincident L323 P5
  constraint midpoint L285 P5
  constraint perpendicular L324 L325
  constraint parallel L324 L326
  constraint parallel L325 L327
  constraint horizontal L324
  constraint coincident L328 P6
  constraint coincident L329 P6
  constraint midpoint L286 P6
  measures "d62" distance of L289.end L290.end
  measures "d63" distance of L288.end L289.end
  measures "d64" distance of L294.end L295.end
  measures "d65" distance of L295.end L296.end
  measures "d66" distance of L301.end L302.end
  measures "d67" distance of L300.end L301.end
  measures "d68" distance of L306.end L307.end
  measures "d69" distance of L307.end L308.end
  measures "d70" distance of L312.end L313.end
  measures "d71" distance of L313.end L314.end
  measures "d72" distance of L318.end L319.end
  measures "d73" distance of L319.end L320.end
  measures "d74" distance of L325.end L326.end
  measures "d75" distance of L324.end L325.end
extrude "Extrusion14" add sketch "Skizze4" against normal blind 6 contours L248 L249 L250 L251 L252 L253 | L254 L255 L256 L257 L258 L259 | L260 L261 L262 L263 L264 L265
extrude "Extrusion15" add sketch "Skizze4" against normal blind 4 contours L180 L181 L182 L183 | L192 L193 L194 L195
extrude "Extrusion16" add sketch "Skizze4" against normal blind 4 contours L168 L169 L170 L171
extrude "Extrusion17" add sketch "Skizze4" against normal blind 3.5 contours L0 L1 L2 L3 | L116 L117 L118 L119 | L120 L121 L122 L123 | L172 L173 L174 L175 | L176 L177 L178 L179 | L184 L185 L186 L187 | L224 L225 L226 L227 | L228 L229 L230 L231
extrude "Extrusion18" add sketch "Skizze4" against normal blind 2 contours L20 L21 L22 L23
extrude "Extrusion19" add sketch "Skizze4" against normal blind 1.7 contours L4 L5 L6 L7 | L8 L9 L10 L11 | L12 L13 L14 L15 | L16 L17 L18 L19 | L24 L25 L26 L27 | L28 L29 L30 L31 | L32 L33 L34 L35 | L36 L37 L38 L39 | L40 L41 L42 L43 | L44 L45 L46 L47 | L48 L49 L50 L51 | L52 L53 L54 L55 | L56 L57 L58 L59 | L60 L61 L62 L63 | L64 L65 L66 L67 | L96 L97 L98 L99 | L100 L101 L102 L103 | L104 L105 L106 L107 | L108 L109 L110 L111 | L112 L113 L114 L115 | L124 L125 L126 L127 | L128 L129 L130 L131 | L132 L133 L134 L135 | L136 L137 L138 L139 | L140 L141 L142 L143 | L144 L145 L146 L147 | L148 L149 L150 L151 | L152 L153 L154 L155 | L156 L157 L158 L159 | L160 L161 L162 L163 | L164 L165 L166 L167 | L200 L201 L202 L203 | L204 L205 L206 L207 | L208 L209 L210 L211 | L212 L213 L214 L215 | L216 L217 L218 L219 | L220 L221 L222 L223 | L232 L233 L234 L235 | L236 L237 L238 L239 | L240 L241 L242 L243 | L244 L245 L246 L247 | L288 L289 L290 L291 | L294 L295 L296 L297 | L300 L301 L302 L303 | L306 L307 L308 L309 | L312 L313 L314 L315 | L318 L319 L320 L321 | L324 L325 L326 L327
extrude "Extrusion20" add sketch "Skizze4" against normal blind 3 contours L274 L275 L276 L277
extrude "Extrusion22" add sketch "Skizze4" against normal blind 1.6 contours L188 L189 L190 L191 | L196 L197 L198 L199
extrude "Extrusion23" add sketch "Skizze1" along normal blind 0.1 contours L154 L155 L156 L157 | L158 L159 L160 L161 | L162 L163 L164 L165
